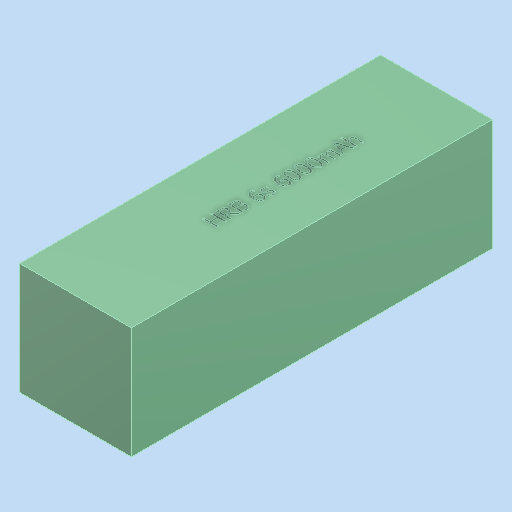
# Autodesk Inventor part: акб
Saved by Autodesk Inventor 2025 (Build 290162000, 162)
## iProperties
Created: 2025-02-20
Part Number: акб
Material: для акб
Document SubType Name: Modeling
Designer: volko
Density: 2.24 g/cm^3
Appearance: Гладкий — темный цвет морской волны
Mass: 799.346 g
Surface Area: 350.955 cm^2
Volume: 356.851 cm^3
Finish1_Area: 11,917 мм^2
Finish1_Appearance: American Cherry
Finish2_Area: 135,021 мм^2
Finish2_Appearance: Black
Author: volko
Autodesk Inventor part; units mm, degrees
ref_plane "YZ Plane" through (0, 0, 0) normal (1, 0, 0) x (0, 1, 0)
ref_plane "XZ Plane" through (0, 0, 0) normal (0, 1, 0) x (-1, 0, 0)
ref_plane "XY Plane" through (0, 0, 0) normal (0, 0, 1) x (1, 0, 0)
sketch "Эскиз1" plane through (0, 0, 0) normal (0, 1, 0) x (-1, 0, 0)
  line L0 (24, 77.5) -> (-24, 77.5)
  line L1 (-24, 77.5) -> (-24, -77.5)
  line L2 (-24, -77.5) -> (24, -77.5)
  line L3 (24, -77.5) -> (24, 77.5)
  line L4 (0, -108.5) -> (0, 108.5) projected
  line L5 (33.6, 0) -> (-33.6, 0) projected
  point P0 (0, 0)
  point P1 (0, 77.5)
  point P2 (24, 0)
  dimension "d0" = 48
  dimension "d1" = 155
  constraints: 8 end point, 2 midpoint, 2 parallel, 2 point on line, 1 horizontal, 1 perpendicular
  measures "d0" distance of L0.start L0.end
  measures "d1" distance of L0.end L1.end
extrude "Выдавливание1" add sketch "Эскиз1" along normal blind 48
sketch "Эскиз2" plane through (0, 48, 0) normal (0, 1, 0) x (1, 0, 0)
  line L0 (-1.5844, -22.3202) -> (-1.5844, 43) construction
  line L1 (-1.5844, 43) -> (4, 43) construction
  line L2 (4, 43) -> (4, -22.3202) construction
  line L3 (4, -22.3202) -> (-1.5844, -22.3202) construction
  line L4 (4.7875, -17.2731) -> (4.7875, -18.0838)
  line L5 (4.7875, -18.0838) -> (1.8017, -18.0838)
  line L6 (1.8017, -18.0838) -> (1.8017, -20.8916)
  line L7 (1.8017, -20.8916) -> (4.7875, -20.8916)
  line L8 (4.7875, -20.8916) -> (4.7875, -21.7023)
  line L9 (4.7875, -21.7023) -> (-1.3125, -21.7023)
  line L10 (-1.3125, -21.7023) -> (-1.3125, -20.8916)
  line L11 (-1.3125, -20.8916) -> (1.08, -20.8916)
  line L12 (1.08, -20.8916) -> (1.08, -18.0838)
  line L13 (1.08, -18.0838) -> (-1.3125, -18.0838)
  line L14 (-1.3125, -18.0838) -> (-1.3125, -17.2731)
  line L15 (-1.3125, -17.2731) -> (4.7875, -17.2731)
  line L16 (4.7875, -11.3164) -> (4.7875, -12.3694)
  line L17 (4.7875, -12.3694) -> (2.3603, -14.2972)
  line L18 (2.3603, -14.2972) -> (2.3603, -15.2266)
  line L19 (2.3603, -15.2266) -> (4.7875, -15.2266)
  line L20 (4.7875, -15.2266) -> (4.7875, -16.0373)
  line L21 (4.7875, -16.0373) -> (-1.3125, -16.0373)
  line L22 (-1.3125, -16.0373) -> (-1.3125, -14.4653)
  spline S0 degree 2 poles (-1.3125, -14.4653) (-1.3125, -13.9413) (-1.1988, -13.2344) (-0.9912, -12.9131) knots 0 0 0 1 2 2 2
  spline S1 degree 2 poles (-0.9912, -12.9131) (-0.7836, -12.5918) (-0.136, -12.2211) (0.3435, -12.2211) knots 0 0 0 1 2 2 2
  spline S2 degree 2 poles (0.3435, -12.2211) (1.0108, -12.2211) (1.9154, -12.9032) (2.1329, -13.4865) knots 0 0 0 1 2 2 2
  line L23 (2.1329, -13.4865) -> (4.7875, -11.3164)
  spline S3 degree 2 poles (0.4077, -13.0664) (0.1408, -13.0664) (-0.2695, -13.2542) (-0.403, -13.4519) knots 0 0 0 1 2 2 2
  spline S4 degree 2 poles (-0.403, -13.4519) (-0.5167, -13.625) (-0.6106, -14.0847) (-0.6106, -14.4208) knots 0 0 0 1 2 2 2
  line L24 (-0.6106, -14.4208) -> (-0.6106, -15.2266)
  line L25 (-0.6106, -15.2266) -> (1.6831, -15.2266)
  line L26 (1.6831, -15.2266) -> (1.6831, -14.5147)
  spline S5 degree 2 poles (1.6831, -14.5147) (1.6831, -14.1638) (1.5595, -13.6052) (1.3667, -13.4124) knots 0 0 0 1 2 2 2
  spline S6 degree 2 poles (1.3667, -13.4124) (1.1987, -13.2344) (0.7241, -13.0664) (0.4077, -13.0664) knots 0 0 0 1 2 2 2
  spline S7 degree 2 poles (2.914, -6.6945) (3.3688, -6.6945) (4.0658, -7.0405) (4.2931, -7.3272) knots 0 0 0 1 2 2 2
  spline S8 degree 2 poles (4.2931, -7.3272) (4.5601, -7.6733) (4.7875, -8.4592) (4.7875, -9.0821) knots 0 0 0 1 2 2 2
  line L27 (4.7875, -9.0821) -> (4.7875, -10.832)
  line L28 (4.7875, -10.832) -> (-1.3125, -10.832)
  line L29 (-1.3125, -10.832) -> (-1.3125, -9.2156)
  spline S9 degree 2 poles (-1.3125, -9.2156) (-1.3125, -8.563) (-1.2285, -7.9105) (-1.0654, -7.6139) knots 0 0 0 1 2 2 2
  spline S10 degree 2 poles (-1.0654, -7.6139) (-0.8924, -7.2827) (-0.3239, -6.9812) (0.0617, -6.9812) knots 0 0 0 1 2 2 2
  spline S11 degree 2 poles (0.0617, -6.9812) (0.4918, -6.9812) (1.1739, -7.436) (1.3667, -7.8364) knots 0 0 0 1 2 2 2
  line L30 (1.3667, -7.8364) -> (1.3964, -7.8364)
  spline S12 degree 2 poles (1.3964, -7.8364) (1.5447, -7.2926) (2.3307, -6.6945) (2.914, -6.6945) knots 0 0 0 1 2 2 2
  spline S13 degree 2 poles (2.9486, -7.5398) (2.6025, -7.5398) (2.1576, -7.7375) (1.9995, -8.0341) knots 0 0 0 1 2 2 2
  spline S14 degree 2 poles (1.9995, -8.0341) (1.9006, -8.2269) (1.8413, -8.6817) (1.8413, -9.1019) knots 0 0 0 1 2 2 2
  line L31 (1.8413, -9.1019) -> (1.8413, -10.0213)
  line L32 (1.8413, -10.0213) -> (4.0954, -10.0213)
  line L33 (4.0954, -10.0213) -> (4.0954, -9.3639)
  spline S15 degree 2 poles (4.0954, -9.3639) (4.0954, -8.83) (3.9965, -8.217) (3.8384, -7.9797) knots 0 0 0 1 2 2 2
  spline S16 degree 2 poles (3.8384, -7.9797) (3.6752, -7.7523) (3.2699, -7.5398) (2.9486, -7.5398) knots 0 0 0 1 2 2 2
  spline S17 degree 2 poles (0.1754, -7.8265) (-0.0421, -7.8265) (-0.3684, -7.9748) (-0.4623, -8.1379) knots 0 0 0 1 2 2 2
  spline S18 degree 2 poles (-0.4623, -8.1379) (-0.571, -8.3357) (-0.6205, -8.8152) (-0.6205, -9.2452) knots 0 0 0 1 2 2 2
  line L34 (-0.6205, -9.2452) -> (-0.6205, -10.0213)
  line L35 (-0.6205, -10.0213) -> (1.1641, -10.0213)
  line L36 (1.1641, -10.0213) -> (1.1641, -9.1019)
  spline S19 degree 2 poles (1.1641, -9.1019) (1.1641, -8.7212) (1.085, -8.3604) (0.9614, -8.1676) knots 0 0 0 1 2 2 2
  spline S20 degree 2 poles (0.9614, -8.1676) (0.8427, -7.9797) (0.4621, -7.8265) (0.1754, -7.8265) knots 0 0 0 1 2 2 2
  spline S21 degree 2 poles (2.8102, 0.4139) (3.2798, 0.4139) (4.0756, 0.1025) (4.3426, -0.1595) knots 0 0 0 1 2 2 2
  spline S22 degree 2 poles (4.3426, -0.1595) (4.6243, -0.4314) (4.916, -1.1135) (4.916, -1.5238) knots 0 0 0 1 2 2 2
  spline S23 degree 2 poles (4.916, -1.5238) (4.916, -1.9341) (4.6392, -2.6113) (4.3623, -2.8684) knots 0 0 0 1 2 2 2
  spline S24 degree 2 poles (4.3623, -2.8684) (4.0311, -3.1848) (2.9189, -3.5407) (2.1082, -3.5407) knots 0 0 0 1 2 2 2
  spline S25 degree 2 poles (2.1082, -3.5407) (1.3123, -3.5407) (0.032, -3.2144) (-0.4425, -2.8733) knots 0 0 0 1 2 2 2
  spline S26 degree 2 poles (-0.4425, -2.8733) (-0.9072, -2.5421) (-1.4262, -1.4942) (-1.4262, -0.807) knots 0 0 0 1 2 2 2
  spline S27 degree 2 poles (-1.4262, -0.807) (-1.4262, -0.6044) (-1.3867, -0.2485) (-1.3422, -0.115) knots 0 0 0 1 2 2 2
  line L37 (-1.3422, -0.115) -> (-0.5562, -0.115)
  line L38 (-0.5562, -0.115) -> (-0.5562, -0.1496)
  spline S28 degree 2 poles (-0.5562, -0.1496) (-0.6155, -0.2633) (-0.7193, -0.6785) (-0.7193, -0.9158) knots 0 0 0 1 2 2 2
  spline S29 degree 2 poles (-0.7193, -0.9158) (-0.7193, -1.6771) (0.3089, -2.6113) (1.3173, -2.7003) knots 0 0 0 1 2 2 2
  spline S30 degree 2 poles (1.3173, -2.7003) (1.1146, -2.4087) (0.8922, -1.7957) (0.8922, -1.4299) knots 0 0 0 1 2 2 2
  spline S31 degree 2 poles (0.8922, -1.4299) (0.8922, -1.074) (1.0355, -0.5401) (1.253, -0.2485) knots 0 0 0 1 2 2 2
  spline S32 degree 2 poles (1.253, -0.2485) (1.5051, 0.0877) (2.2862, 0.4139) (2.8102, 0.4139) knots 0 0 0 1 2 2 2
  spline S33 degree 2 poles (2.8448, -0.4165) (2.4691, -0.4165) (1.9599, -0.6143) (1.782, -0.8318) knots 0 0 0 1 2 2 2
  spline S34 degree 2 poles (1.782, -0.8318) (1.6534, -0.9949) (1.5694, -1.4002) (1.5694, -1.6128) knots 0 0 0 1 2 2 2
  spline S35 degree 2 poles (1.5694, -1.6128) (1.5694, -1.8995) (1.7424, -2.4383) (1.9055, -2.7003) knots 0 0 0 1 2 2 2
  spline S36 degree 2 poles (1.9055, -2.7003) (1.9945, -2.7053) (2.1626, -2.7152) (2.2911, -2.7152) knots 0 0 0 1 2 2 2
  spline S37 degree 2 poles (2.2911, -2.7152) (2.9239, -2.7152) (3.6999, -2.468) (3.9026, -2.2801) knots 0 0 0 1 2 2 2
  spline S38 degree 2 poles (3.9026, -2.2801) (4.0954, -2.1071) (4.2487, -1.7314) (4.2487, -1.5189) knots 0 0 0 1 2 2 2
  spline S39 degree 2 poles (4.2487, -1.5189) (4.2487, -1.0246) (3.5467, -0.4165) (2.8448, -0.4165) knots 0 0 0 1 2 2 2
  spline S40 degree 2 poles (4.8962, 2.4852) (4.8962, 2.0254) (4.6491, 1.2296) (4.5106, 0.9676) knots 0 0 0 1 2 2 2
  line L39 (4.5106, 0.9676) -> (3.6456, 0.9676)
  line L40 (3.6456, 0.9676) -> (3.6456, 1.0071)
  spline S41 degree 2 poles (3.6456, 1.0071) (3.7247, 1.106) (3.9125, 1.3729) (4.0163, 1.5954) knots 0 0 0 1 2 2 2
  spline S42 degree 2 poles (4.0163, 1.5954) (4.1102, 1.7882) (4.2487, 2.2627) (4.2487, 2.5148) knots 0 0 0 1 2 2 2
  spline S43 degree 2 poles (4.2487, 2.5148) (4.2487, 2.6977) (4.1646, 3.1179) (4.0954, 3.2168) knots 0 0 0 1 2 2 2
  spline S44 degree 2 poles (4.0954, 3.2168) (4.0015, 3.3601) (3.7889, 3.4887) (3.5714, 3.4887) knots 0 0 0 1 2 2 2
  spline S45 degree 2 poles (3.5714, 3.4887) (3.2995, 3.4887) (3.0178, 3.1921) (2.9239, 2.8114) knots 0 0 0 1 2 2 2
  spline S46 degree 2 poles (2.9239, 2.8114) (2.8893, 2.6631) (2.7904, 2.1886) (2.736, 1.9859) knots 0 0 0 1 2 2 2
  spline S47 degree 2 poles (2.736, 1.9859) (2.5828, 1.4619) (1.95, 0.9874) (1.5002, 0.9874) knots 0 0 0 1 2 2 2
  spline S48 degree 2 poles (1.5002, 0.9874) (0.8773, 0.9874) (0.1012, 1.9216) (0.1012, 2.6928) knots 0 0 0 1 2 2 2
  spline S49 degree 2 poles (0.1012, 2.6928) (0.1012, 3.0734) (0.2891, 3.8446) (0.4324, 4.1066) knots 0 0 0 1 2 2 2
  line L41 (0.4324, 4.1066) -> (1.258, 4.1066)
  line L42 (1.258, 4.1066) -> (1.258, 4.067)
  spline S50 degree 2 poles (1.258, 4.067) (1.0207, 3.7704) (0.7488, 3.0487) (0.7488, 2.678) knots 0 0 0 1 2 2 2
  spline S51 degree 2 poles (0.7488, 2.678) (0.7488, 2.2973) (1.0701, 1.7733) (1.3914, 1.7733) knots 0 0 0 1 2 2 2
  spline S52 degree 2 poles (1.3914, 1.7733) (1.6831, 1.7733) (1.9649, 2.0848) (2.0538, 2.4308) knots 0 0 0 1 2 2 2
  spline S53 degree 2 poles (2.0538, 2.4308) (2.0983, 2.5989) (2.1873, 3.024) (2.2417, 3.2563) knots 0 0 0 1 2 2 2
  spline S54 degree 2 poles (2.2417, 3.2563) (2.3702, 3.7605) (2.9585, 4.2746) (3.4676, 4.2746) knots 0 0 0 1 2 2 2
  spline S55 degree 2 poles (3.4676, 4.2746) (3.7642, 4.2746) (4.2882, 4.0423) (4.481, 3.8149) knots 0 0 0 1 2 2 2
  spline S56 degree 2 poles (4.481, 3.8149) (4.6837, 3.5727) (4.8962, 2.9548) (4.8962, 2.4852) knots 0 0 0 1 2 2 2
  spline S57 degree 2 poles (2.8102, 11.3534) (3.2798, 11.3534) (4.0756, 11.042) (4.3426, 10.78) knots 0 0 0 1 2 2 2
  spline S58 degree 2 poles (4.3426, 10.78) (4.6243, 10.5081) (4.916, 9.8259) (4.916, 9.4156) knots 0 0 0 1 2 2 2
  spline S59 degree 2 poles (4.916, 9.4156) (4.916, 9.0054) (4.6392, 8.3281) (4.3623, 8.0711) knots 0 0 0 1 2 2 2
  spline S60 degree 2 poles (4.3623, 8.0711) (4.0311, 7.7547) (2.9189, 7.3988) (2.1082, 7.3988) knots 0 0 0 1 2 2 2
  spline S61 degree 2 poles (2.1082, 7.3988) (1.3123, 7.3988) (0.032, 7.725) (-0.4425, 8.0661) knots 0 0 0 1 2 2 2
  spline S62 degree 2 poles (-0.4425, 8.0661) (-0.9072, 8.3973) (-1.4262, 9.4453) (-1.4262, 10.1324) knots 0 0 0 1 2 2 2
  spline S63 degree 2 poles (-1.4262, 10.1324) (-1.4262, 10.3351) (-1.3867, 10.691) (-1.3422, 10.8245) knots 0 0 0 1 2 2 2
  line L43 (-1.3422, 10.8245) -> (-0.5562, 10.8245)
  line L44 (-0.5562, 10.8245) -> (-0.5562, 10.7899)
  spline S64 degree 2 poles (-0.5562, 10.7899) (-0.6155, 10.6762) (-0.7193, 10.2609) (-0.7193, 10.0237) knots 0 0 0 1 2 2 2
  spline S65 degree 2 poles (-0.7193, 10.0237) (-0.7193, 9.2624) (0.3089, 8.3281) (1.3173, 8.2391) knots 0 0 0 1 2 2 2
  spline S66 degree 2 poles (1.3173, 8.2391) (1.1146, 8.5308) (0.8922, 9.1438) (0.8922, 9.5096) knots 0 0 0 1 2 2 2
  spline S67 degree 2 poles (0.8922, 9.5096) (0.8922, 9.8655) (1.0355, 10.3994) (1.253, 10.691) knots 0 0 0 1 2 2 2
  spline S68 degree 2 poles (1.253, 10.691) (1.5051, 11.0271) (2.2862, 11.3534) (2.8102, 11.3534) knots 0 0 0 1 2 2 2
  spline S69 degree 2 poles (2.8448, 10.5229) (2.4691, 10.5229) (1.9599, 10.3252) (1.782, 10.1077) knots 0 0 0 1 2 2 2
  spline S70 degree 2 poles (1.782, 10.1077) (1.6534, 9.9446) (1.5694, 9.5392) (1.5694, 9.3267) knots 0 0 0 1 2 2 2
  spline S71 degree 2 poles (1.5694, 9.3267) (1.5694, 9.04) (1.7424, 8.5011) (1.9055, 8.2391) knots 0 0 0 1 2 2 2
  spline S72 degree 2 poles (1.9055, 8.2391) (1.9945, 8.2342) (2.1626, 8.2243) (2.2911, 8.2243) knots 0 0 0 1 2 2 2
  spline S73 degree 2 poles (2.2911, 8.2243) (2.9239, 8.2243) (3.6999, 8.4715) (3.9026, 8.6593) knots 0 0 0 1 2 2 2
  spline S74 degree 2 poles (3.9026, 8.6593) (4.0954, 8.8323) (4.2487, 9.208) (4.2487, 9.4206) knots 0 0 0 1 2 2 2
  spline S75 degree 2 poles (4.2487, 9.4206) (4.2487, 9.9149) (3.5467, 10.5229) (2.8448, 10.5229) knots 0 0 0 1 2 2 2
  spline S76 degree 2 poles (1.7375, 15.8716) (3.3786, 15.8716) (4.916, 14.9175) (4.916, 13.9239) knots 0 0 0 1 2 2 2
  spline S77 degree 2 poles (4.916, 13.9239) (4.916, 12.9155) (3.349, 11.9713) (1.7424, 11.9713) knots 0 0 0 1 2 2 2
  spline S78 degree 2 poles (1.7424, 11.9713) (0.0914, 11.9713) (-1.4361, 12.9254) (-1.4361, 13.9239) knots 0 0 0 1 2 2 2
  spline S79 degree 2 poles (-1.4361, 13.9239) (-1.4361, 14.9274) (0.1457, 15.8716) (1.7375, 15.8716) knots 0 0 0 1 2 2 2
  spline S80 degree 2 poles (3.5961, 14.8236) (3.2946, 14.9422) (2.3653, 15.0411) (1.7375, 15.0411) knots 0 0 0 1 2 2 2
  spline S81 degree 2 poles (1.7375, 15.0411) (1.1097, 15.0411) (0.1853, 14.9422) (-0.1261, 14.8186) knots 0 0 0 1 2 2 2
  spline S82 degree 2 poles (-0.1261, 14.8186) (-0.4376, 14.6951) (-0.7589, 14.265) (-0.7589, 13.9239) knots 0 0 0 1 2 2 2
  spline S83 degree 2 poles (-0.7589, 13.9239) (-0.7589, 13.5828) (-0.4376, 13.1429) (-0.1163, 13.0143) knots 0 0 0 1 2 2 2
  spline S84 degree 2 poles (-0.1163, 13.0143) (0.1952, 12.8908) (1.1443, 12.8018) (1.7424, 12.8018) knots 0 0 0 1 2 2 2
  spline S85 degree 2 poles (1.7424, 12.8018) (2.385, 12.8018) (3.2452, 12.8809) (3.5813, 13.0094) knots 0 0 0 1 2 2 2
  spline S86 degree 2 poles (3.5813, 13.0094) (3.8977, 13.128) (4.2388, 13.568) (4.2388, 13.9239) knots 0 0 0 1 2 2 2
  spline S87 degree 2 poles (4.2388, 13.9239) (4.2388, 14.2601) (3.9175, 14.7) (3.5961, 14.8236) knots 0 0 0 1 2 2 2
  spline S88 degree 2 poles (1.7375, 20.449) (3.3786, 20.449) (4.916, 19.495) (4.916, 18.5014) knots 0 0 0 1 2 2 2
  spline S89 degree 2 poles (4.916, 18.5014) (4.916, 17.493) (3.349, 16.5488) (1.7424, 16.5488) knots 0 0 0 1 2 2 2
  spline S90 degree 2 poles (1.7424, 16.5488) (0.0914, 16.5488) (-1.4361, 17.5028) (-1.4361, 18.5014) knots 0 0 0 1 2 2 2
  spline S91 degree 2 poles (-1.4361, 18.5014) (-1.4361, 19.5049) (0.1457, 20.449) (1.7375, 20.449) knots 0 0 0 1 2 2 2
  spline S92 degree 2 poles (3.5961, 19.4011) (3.2946, 19.5197) (2.3653, 19.6186) (1.7375, 19.6186) knots 0 0 0 1 2 2 2
  spline S93 degree 2 poles (1.7375, 19.6186) (1.1097, 19.6186) (0.1853, 19.5197) (-0.1261, 19.3961) knots 0 0 0 1 2 2 2
  spline S94 degree 2 poles (-0.1261, 19.3961) (-0.4376, 19.2725) (-0.7589, 18.8425) (-0.7589, 18.5014) knots 0 0 0 1 2 2 2
  spline S95 degree 2 poles (-0.7589, 18.5014) (-0.7589, 18.1603) (-0.4376, 17.7203) (-0.1163, 17.5918) knots 0 0 0 1 2 2 2
  spline S96 degree 2 poles (-0.1163, 17.5918) (0.1952, 17.4682) (1.1443, 17.3793) (1.7424, 17.3793) knots 0 0 0 1 2 2 2
  spline S97 degree 2 poles (1.7424, 17.3793) (2.385, 17.3793) (3.2452, 17.4583) (3.5813, 17.5869) knots 0 0 0 1 2 2 2
  spline S98 degree 2 poles (3.5813, 17.5869) (3.8977, 17.7055) (4.2388, 18.1455) (4.2388, 18.5014) knots 0 0 0 1 2 2 2
  spline S99 degree 2 poles (4.2388, 18.5014) (4.2388, 18.8375) (3.9175, 19.2775) (3.5961, 19.4011) knots 0 0 0 1 2 2 2
  spline S100 degree 2 poles (1.7375, 25.0265) (3.3786, 25.0265) (4.916, 24.0724) (4.916, 23.0789) knots 0 0 0 1 2 2 2
  spline S101 degree 2 poles (4.916, 23.0789) (4.916, 22.0704) (3.349, 21.1263) (1.7424, 21.1263) knots 0 0 0 1 2 2 2
  spline S102 degree 2 poles (1.7424, 21.1263) (0.0914, 21.1263) (-1.4361, 22.0803) (-1.4361, 23.0789) knots 0 0 0 1 2 2 2
  spline S103 degree 2 poles (-1.4361, 23.0789) (-1.4361, 24.0823) (0.1457, 25.0265) (1.7375, 25.0265) knots 0 0 0 1 2 2 2
  spline S104 degree 2 poles (3.5961, 23.9785) (3.2946, 24.0972) (2.3653, 24.196) (1.7375, 24.196) knots 0 0 0 1 2 2 2
  spline S105 degree 2 poles (1.7375, 24.196) (1.1097, 24.196) (0.1853, 24.0972) (-0.1261, 23.9736) knots 0 0 0 1 2 2 2
  spline S106 degree 2 poles (-0.1261, 23.9736) (-0.4376, 23.85) (-0.7589, 23.4199) (-0.7589, 23.0789) knots 0 0 0 1 2 2 2
  spline S107 degree 2 poles (-0.7589, 23.0789) (-0.7589, 22.7378) (-0.4376, 22.2978) (-0.1163, 22.1693) knots 0 0 0 1 2 2 2
  spline S108 degree 2 poles (-0.1163, 22.1693) (0.1952, 22.0457) (1.1443, 21.9567) (1.7424, 21.9567) knots 0 0 0 1 2 2 2
  spline S109 degree 2 poles (1.7424, 21.9567) (2.385, 21.9567) (3.2452, 22.0358) (3.5813, 22.1643) knots 0 0 0 1 2 2 2
  spline S110 degree 2 poles (3.5813, 22.1643) (3.8977, 22.283) (4.2388, 22.7229) (4.2388, 23.0789) knots 0 0 0 1 2 2 2
  spline S111 degree 2 poles (4.2388, 23.0789) (4.2388, 23.415) (3.9175, 23.8549) (3.5961, 23.9785) knots 0 0 0 1 2 2 2
  line L45 (4.7875, 31.1117) -> (2.1379, 31.1117)
  spline S112 degree 2 poles (2.1379, 31.1117) (1.8215, 31.1117) (1.2827, 31.0622) (1.1344, 30.9831) knots 0 0 0 1 2 2 2
  spline S113 degree 2 poles (1.1344, 30.9831) (0.9713, 30.9041) (0.8131, 30.6025) (0.8131, 30.3405) knots 0 0 0 1 2 2 2
  spline S114 degree 2 poles (0.8131, 30.3405) (0.8131, 30.1032) (1.1047, 29.5595) (1.3816, 29.2728) knots 0 0 0 1 2 2 2
  spline S115 degree 2 poles (1.3816, 29.2728) (1.4508, 29.2777) (1.6435, 29.2876) (1.7721, 29.2876) knots 0 0 0 1 2 2 2
  line L46 (1.7721, 29.2876) -> (4.7875, 29.2876)
  line L47 (4.7875, 29.2876) -> (4.7875, 28.5165)
  line L48 (4.7875, 28.5165) -> (2.1379, 28.5165)
  spline S116 degree 2 poles (2.1379, 28.5165) (1.8215, 28.5165) (1.2827, 28.467) (1.1344, 28.3879) knots 0 0 0 1 2 2 2
  spline S117 degree 2 poles (1.1344, 28.3879) (0.9713, 28.3088) (0.8131, 28.0073) (0.8131, 27.7453) knots 0 0 0 1 2 2 2
  spline S118 degree 2 poles (0.8131, 27.7453) (0.8131, 27.4981) (1.1245, 26.9494) (1.3667, 26.6924) knots 0 0 0 1 2 2 2
  line L49 (1.3667, 26.6924) -> (4.7875, 26.6924)
  line L50 (4.7875, 26.6924) -> (4.7875, 25.9212)
  line L51 (4.7875, 25.9212) -> (0.21, 25.9212)
  line L52 (0.21, 25.9212) -> (0.21, 26.6924)
  line L53 (0.21, 26.6924) -> (0.7142, 26.6924)
  spline S119 degree 2 poles (0.7142, 26.6924) (0.4127, 26.9939) (0.0815, 27.5871) (0.0815, 27.943) knots 0 0 0 1 2 2 2
  spline S120 degree 2 poles (0.0815, 27.943) (0.0815, 28.3484) (0.4522, 28.9762) (0.8724, 29.1393) knots 0 0 0 1 2 2 2
  spline S121 degree 2 poles (0.8724, 29.1393) (0.4819, 29.4903) (0.0815, 30.1527) (0.0815, 30.5383) knots 0 0 0 1 2 2 2
  spline S122 degree 2 poles (0.0815, 30.5383) (0.0815, 30.8348) (0.2644, 31.3193) (0.472, 31.4972) knots 0 0 0 1 2 2 2
  spline S123 degree 2 poles (0.472, 31.4972) (0.6796, 31.6801) (1.3025, 31.8828) (1.7721, 31.8828) knots 0 0 0 1 2 2 2
  line L54 (1.7721, 31.8828) -> (4.7875, 31.8828)
  line L55 (4.7875, 31.8828) -> (4.7875, 31.1117)
  line L56 (4.7875, 32.3673) -> (-1.3125, 34.4237)
  line L57 (-1.3125, 34.4237) -> (-1.3125, 35.4222)
  line L58 (-1.3125, 35.4222) -> (4.7875, 37.4786)
  line L59 (4.7875, 37.4786) -> (4.7875, 36.6234)
  line L60 (4.7875, 36.6234) -> (3.082, 36.0698)
  line L61 (3.082, 36.0698) -> (3.082, 33.7415)
  line L62 (3.082, 33.7415) -> (4.7875, 33.1878)
  line L63 (4.7875, 33.1878) -> (4.7875, 32.3673)
  line L64 (2.39, 35.8473) -> (-0.4821, 34.9032)
  line L65 (-0.4821, 34.9032) -> (2.39, 33.9639)
  line L66 (2.39, 33.9639) -> (2.39, 35.8473)
  line L67 (4.7875, 41.5914) -> (4.7875, 40.8203)
  line L68 (4.7875, 40.8203) -> (2.1774, 40.8203)
  spline S124 degree 2 poles (2.1774, 40.8203) (1.8611, 40.8203) (1.3173, 40.7609) (1.1542, 40.672) knots 0 0 0 1 2 2 2
  spline S125 degree 2 poles (1.1542, 40.672) (0.9811, 40.578) (0.8131, 40.2419) (0.8131, 39.9552) knots 0 0 0 1 2 2 2
  spline S126 degree 2 poles (0.8131, 39.9552) (0.8131, 39.6685) (1.1196, 39.0605) (1.3667, 38.7688) knots 0 0 0 1 2 2 2
  line L69 (1.3667, 38.7688) -> (4.7875, 38.7688)
  line L70 (4.7875, 38.7688) -> (4.7875, 37.9977)
  line L71 (4.7875, 37.9977) -> (-1.5844, 37.9977)
  line L72 (-1.5844, 37.9977) -> (-1.5844, 38.7688)
  line L73 (-1.5844, 38.7688) -> (0.7192, 38.7688)
  spline S127 degree 2 poles (0.7192, 38.7688) (0.4077, 39.1148) (0.0815, 39.7822) (0.0815, 40.1579) knots 0 0 0 1 2 2 2
  spline S128 degree 2 poles (0.0815, 40.1579) (0.0815, 40.8301) (0.9713, 41.5914) (1.8166, 41.5914) knots 0 0 0 1 2 2 2
  line L74 (1.8166, 41.5914) -> (4.7875, 41.5914)
  point P0 (0, 0)
  constraints: 2 other
extrude "Выдавливание2" cut sketch "Эскиз2" against normal blind 2
